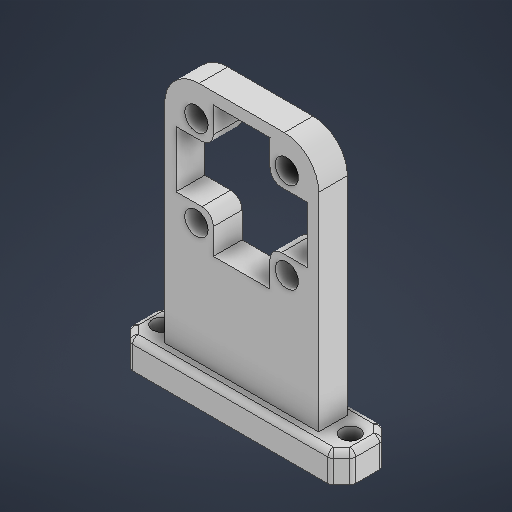
# Autodesk Inventor part: as5600mount_2
Saved by Autodesk Inventor 2025.2 (Build 292293000, 293)
## iProperties
Created: 2025-02-16
Part Number: as5600mount_2
Material: Generic
Document SubType Name: Modeling
Designer: turbo
Density: 1 g/cm^3
Appearance: Default
Author: turbo
Autodesk Inventor part; units mm, degrees
ref_plane "YZ Plane" through (0, 0, 0) normal (1, 0, 0) x (0, 1, 0)
ref_plane "XZ Plane" through (0, 0, 0) normal (0, 1, 0) x (-1, 0, 0)
ref_plane "XY Plane" through (0, 0, 0) normal (0, 0, 1) x (1, 0, 0)
sketch "Sketch1" plane through (0, 0, 0) normal (0, 0, 1) x (1, 0, 0)
  line L0 (0, 0) -> (26.86, 0)
  line L1 (26.86, 0) -> (26.86, 47.18)
  line L2 (26.86, 47.18) -> (0, 47.18)
  line L3 (0, 47.18) -> (0, 0)
  line L4 (2, 38.68) -> (8.5, 38.68)
  line L5 (8.5, 38.68) -> (8.5, 45.18)
  line L6 (8.5, 45.18) -> (18.36, 45.18)
  line L7 (18.36, 45.18) -> (18.36, 38.68)
  line L8 (18.36, 38.68) -> (24.86, 38.68)
  line L9 (24.86, 38.68) -> (24.86, 28.82)
  line L10 (24.86, 28.82) -> (18.36, 28.82)
  line L11 (18.36, 28.82) -> (18.36, 22.32)
  line L12 (18.36, 22.32) -> (8.5, 22.32)
  line L13 (8.5, 22.32) -> (8.5, 28.82)
  line L14 (2, 28.82) -> (2, 38.68)
  line L15 (2, 28.82) -> (8.5, 28.82)
  line L16 (2, 33.75) -> (24.86, 33.75) construction
  line L17 (13.43, 47.18) -> (13.43, 0) construction
  circle A0 centre (5.556, 41.624) radius 2.032
  circle A1 centre (5.556, 25.876) radius 2.032
  circle A2 centre (21.304, 25.876) radius 2.032
  circle A3 centre (21.304, 41.624) radius 2.032
  point P0 (13.43, 33.75)
  point P1 (5.25, 38.68)
  dimension "d0" = 47.18
  dimension "d1" = 26.86
  dimension "d2" = 6.5
  dimension "d3" = 22.86
  dimension "d4" = 2
  dimension "d5" = 4.064
  dimension "d6" = 2.944
  dimension "d7" = 2.944
  constraints: 36 end point, 12 perpendicular, 6 midpoint, 6 point on line, 5 parallel, 4 centre point, 3 equal radius, 3 horizontal, 2 horizontal alignment, 2 vertical alignment, 2 other
  measures "d0" distance of L0.end L1.end
  measures "d1" distance of L0.start L0.end
  measures "d2" distance of L7.end L8.end
  measures "d3" distance between parallel lines of L6 L12
  measures "d4" distance between parallel lines of L2 L6
  measures "d5" diameter of A0
  measures "d6" distance from line of L5 A0.centre
  measures "d7" vertical distance of A0.centre point (5.25, 38.68)
extrude "Extrusion1" add sketch "Sketch1" along normal blind 5
fillet "Fillet1" radius 2 4 edges at (8.5, 28.82, 2.5) (18.36, 28.82, 2.5) (8.5, 38.68, 2.5) (18.36, 38.68, 2.5)
fillet "Fillet2" radius 6 2 edges at (0, 47.18, 2.5) (26.86, 47.18, 2.5)
sketch "Sketch2" plane through (0, 0, 5) normal (0, 0, 1) x (1, 0, 0)
  line L0 (8.5, 45.18) -> (18.36, 45.18) projected
  line L1 (24.86, 38.68) -> (24.86, 28.82) projected
  line L2 (18.36, 22.32) -> (8.5, 22.32) projected
  line L3 (2, 28.82) -> (2, 38.68) projected
  circle A0 centre (13.43, 33.75) radius 11.43
  point P0 (0, 0)
  constraints: 3 tangent, 1 centre point
sketch "Sketch3" plane through (0, 0, 0) normal (0, -1, 0) x (1, 0, 0)
  line L0 (0, 0) -> (26.86, 0) construction
  line L1 (26.86, 0) -> (26.86, 5) construction
  line L2 (0, 5) -> (26.86, 5) construction
  line L3 (0, 0) -> (0, 5) construction
  line L4 (-6, 5) -> (32.86, 5) construction
  line L5 (32.86, 5) -> (32.86, 0)
  line L6 (32.86, 0) -> (-6, 0) construction
  line L7 (-6, 0) -> (-6, 5)
  line L8 (0, 5) -> (26.86, 5) projected
  line L9 (0, 0) -> (26.86, 0) projected
  line L10 (13.43, 5) -> (13.43, 0) construction
  line L11 (13.43, 5) -> (13.43, 0) construction
  circle A0 centre (29.86, 2.5) radius 1.625
  line L12 (26.86, 5) -> (32.86, 0) construction
  circle A1 centre (-3, 2.5) radius 1.625
  line L13 (-6, 0) -> (-4, -2)
  line L14 (-4, -2) -> (30.86, -2)
  line L15 (30.86, -2) -> (32.86, 0)
  line L16 (-6, 5) -> (-4, 7)
  line L17 (-4, 7) -> (30.86, 7)
  line L18 (30.86, 7) -> (32.86, 5)
  line L19 (0, 0) -> (0, 5) projected
  line L20 (0, 5) -> (0, 0)
  line L21 (26.86, 0) -> (26.86, 5) projected
  line L22 (26.86, 5) -> (26.86, 0)
  point P0 (13.43, 2.5)
  dimension "d12" = 6
  dimension "d13" = 3.25
  dimension "d14" = 6
  dimension "d15" = 2
  constraints: 30 end point, 7 midpoint, 4 equal length, 3 parallel, 2 centre point, 2 collinear, 2 horizontal, 2 perpendicular, 2 vertical, 1 coincident, 1 symmetric about line, 1 other
  measures "d12" distance between parallel lines of L5 L1
  measures "d13" diameter of A0
  measures "d14" distance between parallel lines of L3 L7
  measures "d15" distance between parallel lines of L17 L4
extrude "Extrusion2" add sketch "Sketch3" against normal blind 5
fillet "Fillet3" radius 1 16 edges at (13.43, 5, 7) (-6, 5, 2.5) (-5, 5, 6) (-5, 5, -1) (13.43, 5, -2) (31.86, 5, 6) (32.86, 5, 2.5) (31.86, 5, -1) (-6, 2.5, 0) (-6, 2.5, 5) (30.86, 2.5, 7) (-4, 2.5, 7) (32.86, 2.5, 5) (32.86, 2.5, 0) (30.86, 2.5, -2) (-4, 2.5, -2)
body "Solid1"
